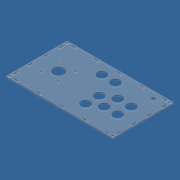
# Autodesk Inventor part: P1704_002
Saved by Autodesk Inventor 2015 SP2 (Build 190223200, 223)
## iProperties
Created: 2017-02-08
Part Number: P1704_002
Project: Manette arcade
Material: Plastique PMMA
Description: Toiture
Document SubType Name: Modeling
Designer: Alexandre.PICOTTE
Authority: 315x180x4
Density: 1.188 g/cm^3
Appearance: Transparent - Clair
Mass: 235.093 g
Surface Area: 1100.65 cm^2
Volume: 197.889 cm^3
Material number: ---
Author: Boris.GAUDARD
Autodesk Inventor part; units mm, degrees
ref_plane "Plan YZ" through (0, 0, 0) normal (1, 0, 0) x (0, 1, 0)
ref_plane "Plan XZ" through (0, 0, 0) normal (0, 1, 0) x (-1, 0, 0)
ref_plane "Plan XY" through (0, 0, 0) normal (0, 0, 1) x (1, 0, 0)
sketch "Esquisse1" plane through (0, 0, 0) normal (0, 0, 1) x (1, 0, 0)
  line L0 (-157.5, 90) -> (157.5, 90)
  line L1 (157.5, 90) -> (157.5, -90)
  line L2 (157.5, -90) -> (-157.5, -90)
  line L3 (-157.5, -90) -> (-157.5, 90)
  line L4 (0, -126) -> (0, 126) construction
  line L5 (-220.5, 0) -> (220.5, 0) construction
  point P0 (0, 0)
  dimension "d0" = 315
  dimension "d1" = 180
  constraints: 8 end point, 2 parallel, 1 horizontal, 1 perpendicular, 2 other
  measures "d0" distance between parallel lines of L1 L3
  measures "d1" distance between parallel lines of L0 L2
extrude "Extrusion1" add sketch "Esquisse1" along normal blind 4
sketch "Esquisse7" plane through (0, 0, 4) normal (0, 0, 1) x (1, 0, 0)
  line L0 (-220.5, 0) -> (220.5, 0) construction
  line L1 (-157.5, 90) -> (-157.5, -90) projected
  point P0 (0, 0)
  point P1 (-92.5, 0)
  dimension "d30" = 65
  dimension "d152" = 0
  measures "d30" distance from line of L1 point (-92.5, 0)
  measures "d152" distance from line of L0 point (-92.5, 0)
hole "Perçage2" at (-92.5, 0, 4) direction (0, 0, -1) diameter 33 end through all
sketch "Esquisse8" plane through (0, 0, 4) normal (0, 0, 1) x (1, 0, 0)
  line L0 (0, -126) -> (0, 126) construction
  line L1 (-220.5, 0) -> (220.5, 0) construction
  line L2 (157.5, 90) -> (-157.5, 90) construction
  point P0 (0, 0)
  point P1 (-20, 55)
  point P2 (20, 55)
  dimension "d38" = 35
  dimension "d39" = 40
  constraints: 1 symmetric about line
  measures "d38" distance from line of L2 point (-20, 55)
  measures "d39" distance of point (20, 55) point (-20, 55)
hole "Perçage3" at (-20, 55, 4) at (20, 55, 4) direction (0, 0, -1) diameter 28 end through all
sketch "Esquisse9" plane through (0, 0, 4) normal (0, 0, 1) x (1, 0, 0)
  line L0 (-142.5, 87) -> (-127.5, 87)
  line L1 (-127.5, 87) -> (-127.5, 83)
  line L2 (-127.5, 83) -> (-142.5, 83)
  line L3 (-142.5, 83) -> (-142.5, 87)
  line L4 (157.5, 90) -> (-157.5, 90) projected
  line L5 (-157.5, 90) -> (-157.5, -90) projected
  line L6 (-220.5, 0) -> (220.5, 0) construction
  line L7 (-75, 87) -> (-60, 87)
  line L8 (-60, 87) -> (-60, 83)
  line L9 (-60, 83) -> (-75, 83)
  line L10 (-75, 83) -> (-75, 87)
  line L11 (-7.5, 87) -> (7.5, 87)
  line L12 (7.5, 87) -> (7.5, 83)
  line L13 (7.5, 83) -> (-7.5, 83)
  line L14 (-7.5, 83) -> (-7.5, 87)
  line L15 (60, 87) -> (75, 87)
  line L16 (75, 87) -> (75, 83)
  line L17 (75, 83) -> (60, 83)
  line L18 (60, 83) -> (60, 87)
  line L19 (127.5, 87) -> (142.5, 87)
  line L20 (142.5, 87) -> (142.5, 83)
  line L21 (142.5, 83) -> (127.5, 83)
  line L22 (127.5, 83) -> (127.5, 87)
  line L23 (-142.5, -87) -> (-127.5, -87)
  line L24 (-127.5, -87) -> (-127.5, -83)
  line L25 (-127.5, -83) -> (-142.5, -83)
  line L26 (-142.5, -83) -> (-142.5, -87)
  line L27 (-75, -87) -> (-60, -87)
  line L28 (-60, -87) -> (-60, -83)
  line L29 (-60, -83) -> (-75, -83)
  line L30 (-75, -83) -> (-75, -87)
  line L31 (-7.5, -87) -> (7.5, -87)
  line L32 (7.5, -87) -> (7.5, -83)
  line L33 (7.5, -83) -> (-7.5, -83)
  line L34 (-7.5, -83) -> (-7.5, -87)
  line L35 (60, -87) -> (75, -87)
  line L36 (75, -87) -> (75, -83)
  line L37 (75, -83) -> (60, -83)
  line L38 (60, -83) -> (60, -87)
  line L39 (127.5, -87) -> (142.5, -87)
  line L40 (142.5, -87) -> (142.5, -83)
  line L41 (142.5, -83) -> (127.5, -83)
  line L42 (127.5, -83) -> (127.5, -87)
  line L43 (0, -126) -> (0, 126) construction
  point P0 (0, 0)
  dimension "d48" = 15
  dimension "d49" = 4
  dimension "d50" = 3
  dimension "d51" = 15
  dimension "d54" = 67.5
  constraints: 80 end point, 20 symmetric about line, 2 horizontal, 2 parallel, 1 perpendicular, 32 other
  measures "d48" distance between parallel lines of L1 L3
  measures "d49" distance between parallel lines of L0 L2
  measures "d50" distance between parallel lines of L4 L0
  measures "d51" distance between parallel lines of L3 L5
  measures "d54" distance of L0.start L7.start
extrude "Extrusion2" cut sketch "Esquisse9" against normal through all
sketch "Esquisse10" plane through (0, 0, 4) normal (0, 0, 1) x (1, 0, 0)
  line L0 (0, -126) -> (0, 126) construction
  line L1 (-220.5, 0) -> (220.5, 0) construction
  line L2 (157.5, 90) -> (-157.5, 90) construction
  line L3 (-157.5, 90) -> (-157.5, -90) construction
  point P0 (0, 0)
  point P1 (-152.5, 85)
  point P2 (152.5, 85)
  point P3 (-152.5, -85)
  point P4 (152.5, -85)
  dimension "d165" = 5
  dimension "d166" = 5
  constraints: 3 symmetric about line
  measures "d165" distance from line of L2 point (-152.5, 85)
  measures "d166" distance from line of L3 point (-152.5, 85)
hole "Perçage4" at (-152.5, 85, 4) at (152.5, 85, 4) at (-152.5, -85, 4) at (152.5, -85, 4) direction (0, 0, -1) diameter 3.2 end through all
sketch "Esquisse11" plane through (0, 0, 4) normal (0, 0, 1) x (1, 0, 0)
  line L0 (-154.5, 75) -> (-150.5, 75)
  line L1 (-150.5, 75) -> (-150.5, 60)
  line L2 (-150.5, 60) -> (-154.5, 60)
  line L3 (-154.5, 60) -> (-154.5, 75)
  line L4 (-157.5, 90) -> (-157.5, -90) projected
  line L5 (157.5, 90) -> (-157.5, 90) projected
  line L6 (0, -126) -> (0, 126) construction
  line L7 (-308.7, 0) -> (308.7, 0) construction
  line L8 (-154.5, 30) -> (-150.5, 30)
  line L9 (-150.5, 30) -> (-150.5, 15)
  line L10 (-150.5, 15) -> (-154.5, 15)
  line L11 (-154.5, 15) -> (-154.5, 30)
  line L12 (-154.5, -15) -> (-150.5, -15)
  line L13 (-150.5, -15) -> (-150.5, -30)
  line L14 (-150.5, -30) -> (-154.5, -30)
  line L15 (-154.5, -30) -> (-154.5, -15)
  line L16 (-154.5, -60) -> (-150.5, -60)
  line L17 (-150.5, -60) -> (-150.5, -75)
  line L18 (-150.5, -75) -> (-154.5, -75)
  line L19 (-154.5, -75) -> (-154.5, -60)
  line L20 (154.5, 75) -> (150.5, 75)
  line L21 (150.5, 75) -> (150.5, 60)
  line L22 (150.5, 60) -> (154.5, 60)
  line L23 (154.5, 60) -> (154.5, 75)
  line L24 (308.7, 0) -> (-308.7, 0) construction
  line L25 (154.5, 30) -> (150.5, 30)
  line L26 (150.5, 30) -> (150.5, 15)
  line L27 (150.5, 15) -> (154.5, 15)
  line L28 (154.5, 15) -> (154.5, 30)
  line L29 (154.5, -15) -> (150.5, -15)
  line L30 (150.5, -15) -> (150.5, -30)
  line L31 (150.5, -30) -> (154.5, -30)
  line L32 (154.5, -30) -> (154.5, -15)
  line L33 (154.5, -60) -> (150.5, -60)
  line L34 (150.5, -60) -> (150.5, -75)
  line L35 (150.5, -75) -> (154.5, -75)
  line L36 (154.5, -75) -> (154.5, -60)
  point P0 (0, 0)
  dimension "d78" = 4
  dimension "d79" = 15
  dimension "d80" = 3
  dimension "d81" = 15
  dimension "d84" = 45
  constraints: 66 end point, 18 symmetric about line, 2 parallel, 1 horizontal, 1 perpendicular, 1 vertical, 24 other
  measures "d78" distance between parallel lines of L1 L3
  measures "d79" distance between parallel lines of L2 L0
  measures "d80" distance between parallel lines of L3 L4
  measures "d81" distance between parallel lines of L5 L0
  measures "d84" distance of L0.start L8.start
extrude "Extrusion3" cut sketch "Esquisse11" against normal through all
sketch "Esquisse12" plane through (0, 0, 4) normal (0, 0, 1) x (1, 0, 0)
  point P0 (0, 0)
  point P1 (-142.5, 83)
  point P2 (-142.5, 87)
  point P3 (-127.5, 87)
  point P4 (-127.5, 83)
  point P5 (-150.5, 75)
  point P6 (-154.5, 75)
  point P7 (-154.5, 60)
  point P8 (-150.5, 60)
  point P9 (-75, 83)
  point P10 (-60, 83)
  point P11 (-60, 87)
  point P12 (-75, 87)
  point P13 (-7.5, 87)
  point P14 (-7.5, 83)
  point P15 (7.5, 87)
  point P16 (60, 87)
  point P17 (60, 83)
  point P18 (75, 83)
  point P19 (75, 87)
  point P20 (142.5, 87)
  point P21 (142.5, 83)
  point P22 (127.5, 83)
  point P23 (127.5, 87)
  point P24 (150.5, 75)
  point P25 (150.5, 60)
  point P26 (154.5, 60)
  point P27 (154.5, 30)
  point P28 (150.5, 30)
  point P29 (154.5, 15)
  point P30 (150.5, 15)
  point P31 (154.5, -60)
  point P32 (150.5, -60)
  point P33 (154.5, -30)
  point P34 (150.5, -30)
  point P35 (150.5, -15)
  point P36 (154.5, -15)
  point P37 (154.5, -75)
  point P38 (150.5, -75)
  point P39 (127.5, -87)
  point P40 (127.5, -83)
  point P41 (142.5, -83)
  point P42 (60, -87)
  point P43 (75, -87)
  point P44 (75, -83)
  point P45 (60, -83)
  point P46 (-7.5, -87)
  point P47 (-7.5, -83)
  point P48 (7.5, -83)
  point P49 (-75, -83)
  point P50 (-60, -83)
  point P51 (-60, -87)
  point P52 (-142.5, -87)
  point P53 (-127.5, -87)
  point P54 (-127.5, -83)
  point P55 (-142.5, -83)
  point P56 (-154.5, -75)
  point P57 (-154.5, -60)
  point P58 (-150.5, -60)
  point P59 (-150.5, 15)
  point P60 (-154.5, 15)
  point P61 (-150.5, -30)
  point P62 (-154.5, -30)
  point P63 (-154.5, -15)
  point P64 (-150.5, -15)
  point P65 (-150.5, 30)
  point P66 (-154.5, 30)
  point P67 (142.5, -87)
  point P68 (154.5, 75)
  point P69 (-75, -87)
  point P70 (7.5, -87)
  point P71 (-150.5, -75)
  point P72 (7.5, 83)
hole "Perçage5" at (-142.5, 83, 4) at (-142.5, 87, 4) at (-127.5, 87, 4) at (-127.5, 83, 4) at (-150.5, 75, 4) at (-154.5, 75, 4) at (-154.5, 60, 4) at (-150.5, 60, 4) at (-75, 83, 4) at (-60, 83, 4) at (-60, 87, 4) at (-75, 87, 4) at (-7.5, 87, 4) at (-7.5, 83, 4) at (7.5, 87, 4) at (60, 87, 4) at (60, 83, 4) at (75, 83, 4) at (75, 87, 4) at (142.5, 87, 4) at (142.5, 83, 4) at (127.5, 83, 4) at (127.5, 87, 4) at (150.5, 75, 4) at (150.5, 60, 4) at (154.5, 60, 4) at (154.5, 30, 4) at (150.5, 30, 4) at (154.5, 15, 4) at (150.5, 15, 4) at (154.5, -60, 4) at (150.5, -60, 4) at (154.5, -30, 4) at (150.5, -30, 4) at (150.5, -15, 4) at (154.5, -15, 4) at (154.5, -75, 4) at (150.5, -75, 4) at (127.5, -87, 4) at (127.5, -83, 4) at (142.5, -83, 4) at (60, -87, 4) at (75, -87, 4) at (75, -83, 4) at (60, -83, 4) at (-7.5, -87, 4) at (-7.5, -83, 4) at (7.5, -83, 4) at (-75, -83, 4) at (-60, -83, 4) direction (0, 0, -1) diameter 1 end through all and at (-60, -87, 4) (-142.5, -87, 4) (-127.5, -87, 4) (-127.5, -83, 4) (-142.5, -83, 4) (-154.5, -75, 4) (-154.5, -60, 4) (-150.5, -60, 4) (-150.5, 15, 4) (-154.5, 15, 4) (-150.5, -30, 4) (-154.5, -30, 4) (-154.5, -15, 4) (-150.5, -15, 4) (-150.5, 30, 4) (-154.5, 30, 4) (142.5, -87, 4) (154.5, 75, 4) (-75, -87, 4) (7.5, -87, 4) (-150.5, -75, 4) (7.5, 83, 4)
chamfer "Chanfrein1" distance 2 angle 45 4 edges at (-157.5, -90, 2) (-157.5, 90, 2) (157.5, 90, 2) (157.5, -90, 2)
sketch "Esquisse13" plane through (0, 0, 4) normal (0, 0, 1) x (1, 0, 0)
  line L0 (-220.5, 0) -> (220.5, 0) construction
  line L1 (0, -126) -> (0, 126) construction
  line L2 (-157.5, 88) -> (-157.5, -88) construction
  line L3 (155.5, 90) -> (-155.5, 90) construction
  point P0 (0, 0)
  point P1 (-117.5, 25)
  point P2 (-67.5, 25)
  point P3 (-117.5, -25)
  point P4 (-67.5, -25)
  dimension "d103" = 50
  dimension "d106" = 50
  dimension "d109" = 40
  dimension "d110" = 65
  constraints: 1 horizontal, 1 vertical, 3 other
  measures "d103" distance of point (-117.5, 25) point (-67.5, 25)
  measures "d106" distance of point (-117.5, 25) point (-117.5, -25)
  measures "d109" distance from line of L2 point (-117.5, 25)
  measures "d110" distance from line of L3 point (-117.5, 25)
hole "Perçage6" at (-117.5, 25, 4) at (-67.5, 25, 4) at (-117.5, -25, 4) at (-67.5, -25, 4) direction (0, 0, -1) diameter 4.5 end through all
sketch "Esquisse15" plane through (0, 0, 4) normal (0, 0, 1) x (1, 0, 0)
  line L0 (-7, -83) -> (7, -83) projected
  line L1 (0, -1924.309) -> (0, 425.7182) construction
  line L2 (-602.5195, 0) -> (602.5195, 0) construction
  circle A0 centre (30, -43) radius 14
  circle A1 centre (30, -3) radius 14
  circle A2 centre (65, 17) radius 14
  circle A3 centre (105, 17) radius 14
  circle A4 centre (65, -23) radius 14
  circle A5 centre (105, -23) radius 14
  line L3 (150.5, -29.5) -> (150.5, -15.5) projected
  line L4 (150.5, 15.5) -> (150.5, 29.5) projected
  dimension "d126" = 28
  dimension "d127" = 28
  dimension "d128" = 40
  dimension "d129" = 20
  dimension "d130" = 35
  dimension "d131" = 28
  dimension "d132" = 40
  dimension "d133" = 28
  dimension "d134" = 28
  dimension "d135" = 35
  dimension "d136" = 20
  dimension "d137" = 28
  dimension "d138" = 40
  dimension "d139" = 40
  dimension "d141" = 30
  dimension "d149" = 40
  dimension "d150" = 20
  dimension "d151" = 30
  constraints: 6 centre point
  measures "d126" diameter of A0
  measures "d127" diameter of A1
  measures "d128" distance of A0.centre A1.centre
  measures "d129" vertical distance of A1.centre A2.centre
  measures "d130" horizontal distance of A1.centre A2.centre
  measures "d131" diameter of A2
  measures "d132" distance of A2.centre A3.centre
  measures "d133" diameter of A3
  measures "d134" diameter of A4
  measures "d135" horizontal distance of A4.centre A0.centre
  measures "d136" vertical distance of A0.centre A4.centre
  measures "d137" diameter of A5
  measures "d138" distance of A4.centre A5.centre
  measures "d139" distance from line of L0 A0.centre
  measures "d141" distance from line of A1.centre L1
  measures "d149" distance of A5.centre A3.centre
  measures "d150" vertical distance of A5.centre A0.centre
  measures "d151" distance from line of L1 A0.centre
extrude "Extrusion4" cut sketch "Esquisse15" against normal blind 10
sketch "Esquisse16" plane through (0, 0, 4) normal (0, 0, 1) x (1, 0, 0)
  line L0 (155.5, 90) -> (-155.5, 90) projected
  line L1 (157.5, -88) -> (157.5, 88) projected
  point P0 (0, 0)
  point P1 (117.5, 70)
  dimension "d156" = 40
  dimension "d157" = 20
  measures "d156" distance from line of L1 point (117.5, 70)
  measures "d157" distance from line of L0 point (117.5, 70)
hole "Perçage7" at (117.5, 70, 4) direction (0, 0, -1) diameter 12 end through all
sketch "Esquisse18" plane through (0, 0, 4) normal (0, 0, 1) x (1, 0, 0)
  circle A0 centre (-152.5, -85) radius 1.6 projected
  circle A1 centre (-152.5, -85) radius 3.25
  circle A2 centre (-152.5, 85) radius 1.6 projected
  circle A3 centre (-152.5, 85) radius 3.25
  circle A4 centre (152.5, 85) radius 1.6 projected
  circle A5 centre (152.5, 85) radius 3.25
  circle A6 centre (152.5, -85) radius 1.6 projected
  circle A7 centre (152.5, -85) radius 3.25
  line L0 (0, -126) -> (0, 126) construction
  line L1 (-220.5, 0) -> (220.5, 0) construction
  point P0 (0, 0)
  dimension "d167" = 6.5
  constraints: 4 centre point, 4 coincident, 3 other
  measures "d167" diameter of A1
extrude "Extrusion5" cut sketch "Esquisse18" against normal blind 2.8
chamfer "Chanfrein2" distance 2 angle 45 4 edges at (-117.5, -22.75, 4) (-117.5, 27.25, 4) (-67.5, 27.25, 4) (-67.5, -22.75, 4)
